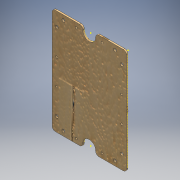
# Autodesk Inventor part: base
Saved by Autodesk Inventor 2016 (Build 200138000, 138)
## iProperties
Created: 2022-06-29
Part Number: base
Material: Generic
Document SubType Name: Modeling
Designer: Teemu S.
Density: 1 g/cm^3
Appearance: Natural Maple - Classic Unfinished
width: 204,250 mm
height: 144,250 mm
stencilW: 180,250 mm
stencilH: 120,250 mm
pinD: 6,000 mm
kerf: 0,075 mm
cornerW: 15,000 mm
cornerH: 10,000 mm
fingerW: 25,000 mm
Author: Teemu S.
Autodesk Inventor part; units mm, degrees
ref_plane "YZ Plane" through (0, 0, 0) normal (1, 0, 0) x (0, 1, 0)
ref_plane "XZ Plane" through (0, 0, 0) normal (0, 1, 0) x (-1, 0, 0)
ref_plane "XY Plane" through (0, 0, 0) normal (0, 0, 1) x (1, 0, 0)
sketch "Sketch1" plane through (0, 0, 0) normal (0, 1, 0) x (-1, 0, 0)
  line L0 (0, 0) -> (144.25, 0)
  line L1 (144.25, 0) -> (144.25, -204.25)
  line L2 (144.25, -204.25) -> (0, -204.25)
  line L3 (0, -204.25) -> (0, 0)
  line L4 (132.25, -12) -> (12, -12) construction
  line L5 (12, -12) -> (12, -192.25) construction
  line L6 (12, -192.25) -> (132.25, -192.25) construction
  line L7 (132.25, -192.25) -> (132.25, -12) construction
  circle A0 centre (135.25, -27) radius 3 construction
  circle A1 centre (122.25, -9) radius 3 construction
  circle A2 centre (122.25, -9) radius 2.925
  circle A3 centre (135.25, -27) radius 2.925
  circle A4 centre (135.25, -177.25) radius 3 construction
  circle A5 centre (122.25, -195.25) radius 3 construction
  circle A6 centre (22, -195.25) radius 3 construction
  circle A7 centre (9, -177.25) radius 3 construction
  circle A8 centre (22, -195.25) radius 2.925
  circle A9 centre (9, -177.25) radius 2.925
  circle A10 centre (135.25, -177.25) radius 2.925
  circle A11 centre (122.25, -195.25) radius 2.925
  circle A12 centre (22, -9) radius 3 construction
  circle A13 centre (9, -27) radius 3 construction
  circle A14 centre (22, -9) radius 2.925
  circle A15 centre (9, -27) radius 2.925
  point P0 (144.25, -102.125)
  point P1 (132.25, -102.125)
  point P2 (72.125, -12)
  point P3 (72.125, 0)
  dimension "width" = 204.25
  dimension "height" = 144.25
  dimension "stencilW" = 180.25
  dimension "stencilH" = 120.25
  dimension "d14" = 6
  dimension "d15" = 6
  dimension "kerf" = 0.075
  dimension "d17" = 0.075
  dimension "cornerW" = 15
  dimension "cornerH" = 10
  dimension "d20" = 6
  dimension "d21" = 6
  dimension "d22" = 6
  dimension "d23" = 6
  dimension "d24" = 10
  dimension "d25" = 15
  dimension "d26" = 10
  dimension "d27" = 15
  dimension "d28" = 0.075
  dimension "d29" = 0.075
  dimension "d30" = 0.075
  dimension "d31" = 0.075
  dimension "d32" = 6
  dimension "d33" = 6
  dimension "d34" = 15
  dimension "d35" = 10
  dimension "d36" = 0.075
  dimension "d37" = 0.075
  constraints: 16 centre point, 16 end point, 8 coincident, 8 tangent, 4 midpoint, 4 parallel, 2 horizontal, 2 perpendicular, 1 horizontal alignment, 1 vertical alignment
  measures "width" distance of L0.end L1.end
  measures "height" distance of L1.end L2.end
  measures "stencilW" distance of L6.end L4.start
  measures "stencilH" distance of L4.start L4.end
  measures "d14" diameter of A0
  measures "d15" diameter of A1
  measures "kerf" radial gap between concentric circles of A0 A3
  measures "d17" radial gap between concentric circles of A1 A2
  measures "cornerW" distance from line of A0.centre L4
  measures "cornerH" distance from line of L7 A1.centre
  measures "d20" diameter of A4
  measures "d21" diameter of A5
  measures "d22" diameter of A6
  measures "d23" diameter of A7
  measures "d24" horizontal distance of A6.centre L5.end
  measures "d25" vertical distance of L5.end A7.centre
  measures "d26" horizontal distance of L6.end A5.centre
  measures "d27" vertical distance of A4.centre L6.end
  measures "d28" radial gap between concentric circles of A4 A10
  measures "d29" radial gap between concentric circles of A5 A11
  measures "d30" radial gap between concentric circles of A6 A8
  measures "d31" radial gap between concentric circles of A7 A9
  measures "d32" diameter of A12
  measures "d33" diameter of A13
  measures "d34" vertical distance of A13.centre L4.end
  measures "d35" horizontal distance of A12.centre L4.end
  measures "d36" radial gap between concentric circles of A12 A14
  measures "d37" radial gap between concentric circles of A13 A15
extrude "Extrusion1" add sketch "Sketch1" along normal blind 3
fillet "Fillet1" radius 6 4 edges at (0, 1.5, 0) (-144.25, 1.5, 0) (0, 1.5, -204.25) (-144.25, 1.5, -204.25)
sketch "Sketch2" plane through (0, 3, 0) normal (0, 1, 0) x (1, 0, 0)
  line L0 (-72.125, -7.125) -> (-72.125, 7.125) construction
  line L1 (-6, 0) -> (-138.25, 0) projected
  line L2 (-59.625, -7.125) -> (-59.625, 7.125)
  line L3 (-84.625, 7.125) -> (-84.625, -7.125)
  arc A0 (-84.625, -7.125) -> (-59.625, -7.125) centre (-72.125, -7.125) ccw
  arc A1 (-59.625, 7.125) -> (-84.625, 7.125) centre (-72.125, 7.125) ccw
  line L4 (-72.125, 0) -> (-57.875, 0) construction
  line L5 (-144.25, 198.25) -> (-144.25, 6) construction
  line L6 (-144.25, 102.125) -> (0, 102.125) construction
  line L7 (0, 6) -> (0, 198.25) construction
  line L8 (-72.125, 211.375) -> (-72.125, 197.125) construction
  line L9 (-59.625, 211.375) -> (-59.625, 197.125)
  line L10 (-84.625, 197.125) -> (-84.625, 211.375)
  arc A2 (-59.625, 211.375) -> (-84.625, 211.375) centre (-72.125, 211.375) ccw
  arc A3 (-84.625, 197.125) -> (-59.625, 197.125) centre (-72.125, 197.125) ccw
  line L11 (-100.1727, 19.625) -> (-55, 19.625) construction
  line L12 (-92.5099, 184.625) -> (-51.3219, 184.625) construction
  point P0 (0, 0)
  dimension "d42" = 90
  dimension "fingerW" = 25
  dimension "d47" = 165
  constraints: 24 end point, 8 point on circle, 6 symmetric about line, 6 tangent, 4 centre point, 4 midpoint, 3 horizontal, 1 parallel, 1 perpendicular, 1 vertical, 2 other
  measures "d42" angle of L4 L0
  measures "fingerW" diameter of A1
  measures "d47" distance between parallel lines of L12 L11
extrude "Extrusion2" cut sketch "Sketch2" against normal blind 3
fillet "Fillet2" radius 6 4 edges at (-84.625, 1.5, 0) (-59.625, 1.5, 0) (-84.625, 1.5, -204.25) (-59.625, 1.5, -204.25)
sketch "Sketch3" plane through (0, 3, 0) normal (0, 1, 0) x (1, 0, 0)
  arc A0 (-59.625, 7.125) -> (-84.625, 7.125) centre (-72.125, 7.125) ccw construction
  arc A1 (-84.625, 197.125) -> (-59.625, 197.125) centre (-72.125, 197.125) ccw construction
  line L0 (-144.25, 198.25) -> (-144.25, 6) construction
  line L1 (0, 6) -> (0, 198.25) construction
  arc A2 (-59.625, 7.125) -> (-84.625, 7.125) centre (-72.125, 7.125) ccw construction
  line L2 (-72.125, 19.625) -> (-72.125, 184.625)
  line L3 (-144.25, 102.125) -> (0, 102.125)
  point P0 (0, 0)
  constraints: 4 end point, 3 point on circle, 2 midpoint
sketch "Sketch4" plane through (0, 3, 0) normal (0, 1, 0) x (1, 0, 0)
  circle A0 centre (-135.25, 77.0833) radius 2
  circle A1 centre (-135.25, 127.1667) radius 2
  arc A2 (-53.625, 204.25) -> (-59.625, 198.25) centre (-53.625, 198.25) ccw construction
  line L0 (-59.625, 198.25) -> (-59.625, 197.125) construction
  arc A3 (-84.625, 197.125) -> (-59.625, 197.125) centre (-72.125, 197.125) ccw construction
  line L1 (-84.625, 197.125) -> (-84.625, 198.25) construction
  arc A4 (-84.625, 198.25) -> (-90.625, 204.25) centre (-90.625, 198.25) ccw construction
  line L2 (-90.625, 204.25) -> (-138.25, 204.25) construction
  arc A5 (-138.25, 204.25) -> (-144.25, 198.25) centre (-138.25, 198.25) ccw construction
  line L3 (-144.25, 198.25) -> (-144.25, 6) construction
  arc A6 (-144.25, 6) -> (-138.25, 0) centre (-138.25, 6) ccw construction
  line L4 (-138.25, 0) -> (-90.625, 0) construction
  arc A7 (-90.625, 0) -> (-84.625, 6) centre (-90.625, 6) ccw construction
  line L5 (-84.625, 6) -> (-84.625, 7.125) construction
  arc A8 (-59.625, 7.125) -> (-84.625, 7.125) centre (-72.125, 7.125) ccw construction
  line L6 (-59.625, 7.125) -> (-59.625, 6) construction
  arc A9 (-59.625, 6) -> (-53.625, 0) centre (-53.625, 6) ccw construction
  line L7 (-53.625, 0) -> (-6, 0) construction
  arc A10 (-6, 0) -> (0, 6) centre (-6, 6) ccw construction
  line L8 (0, 6) -> (0, 198.25) construction
  arc A11 (0, 198.25) -> (-6, 204.25) centre (-6, 198.25) ccw construction
  line L9 (-6, 204.25) -> (-53.625, 204.25) construction
  circle A12 centre (-9, 27) radius 2.925 construction
  circle A13 centre (-22, 9) radius 2.925 construction
  circle A14 centre (-122.25, 195.25) radius 2.925 construction
  circle A15 centre (-135.25, 177.25) radius 2.925 construction
  circle A16 centre (-9, 177.25) radius 2.925 construction
  circle A17 centre (-22, 195.25) radius 2.925 construction
  circle A18 centre (-135.25, 27) radius 2.925 construction
  circle A19 centre (-122.25, 9) radius 2.925 construction
  circle A20 centre (-9, 77.0833) radius 2
  circle A21 centre (-9, 127.1667) radius 2
  circle A22 centre (-97.125, 9) radius 2
  circle A23 centre (-47.125, 9) radius 2
  circle A24 centre (-47.125, 195.25) radius 2
  circle A25 centre (-97.125, 195.25) radius 2
  point P0 (0, 0)
  dimension "d48" = 4
  dimension "d49" = 4
  dimension "d50" = 50.0833
  dimension "d51" = 50.0833
  dimension "d52" = 50.0833
  dimension "d53" = 4
  dimension "d54" = 4
  dimension "d55" = 4
  dimension "d56" = 4
  dimension "d57" = 4
  dimension "d58" = 4
  dimension "d59" = 50
  dimension "d60" = 25.125
  dimension "d61" = 25.125
  constraints: 8 centre point, 6 horizontal alignment, 6 vertical alignment
  measures "d48" diameter of A0
  measures "d49" diameter of A1
  measures "d50" distance of A0.centre A18.centre
  measures "d51" distance of A1.centre A0.centre
  measures "d52" distance of A15.centre A1.centre
  measures "d53" diameter of A20
  measures "d54" diameter of A21
  measures "d55" diameter of A22
  measures "d56" diameter of A23
  measures "d57" diameter of A24
  measures "d58" diameter of A25
  measures "d59" distance of A23.centre A22.centre
  measures "d60" distance of A23.centre A13.centre
  measures "d61" distance of A19.centre A22.centre
extrude "Extrusion3" cut sketch "Sketch4" against normal blind 3
equation "\"width\" = stencilW + 4 * pinD"
equation "\"height\" = stencilH + 4 * pinD"
equation "\"d14\" = pinD"
equation "\"d15\" = pinD"
equation "\"d17\" = kerf"
equation "\"d20\" = pinD"
equation "\"d21\" = pinD"
equation "\"d22\" = pinD"
equation "\"d23\" = pinD"
equation "\"d24\" = cornerH"
equation "\"d25\" = cornerW"
equation "\"d26\" = cornerH"
equation "\"d27\" = cornerW"
equation "\"d28\" = kerf"
equation "\"d29\" = kerf"
equation "\"d30\" = kerf"
equation "\"d31\" = kerf"
equation "\"d32\" = pinD"
equation "\"d33\" = pinD"
equation "\"d34\" = cornerW"
equation "\"d35\" = cornerH"
equation "\"d36\" = kerf"
equation "\"d37\" = kerf"
equation "\"d40\" = pinD"
equation "\"d46\" = pinD"
equation "\"d50\" = d52"
equation "\"d51\" = d50"
equation "\"d60\" = d61"
equation "\"pinD\" = 6"
body "Solid1"
